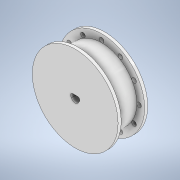
# Autodesk Inventor part: WinderSpoolTraditionalMachining
Saved by Autodesk Inventor 2021 (Build 250183000, 183)
## iProperties
Created: 2020-03-14
Part Number: WinderSpoolTraditionalMachining
Material: Generic
Document SubType Name: Modeling
Designer: elmar
Density: 1 g/cm^3
Appearance: White
Author: elmar
Autodesk Inventor part; units mm, degrees
ref_plane "YZ Plane" through (0, 0, 0) normal (1, 0, 0) x (0, 1, 0)
ref_plane "XZ Plane" through (0, 0, 0) normal (0, 1, 0) x (-1, 0, 0)
ref_plane "XY Plane" through (0, 0, 0) normal (0, 0, 1) x (1, 0, 0)
sketch "Sketch1" plane through (0, 0, 0) normal (0, 0, 1) x (1, 0, 0)
  circle A0 centre (0, 0) radius 22.5
  dimension "d0" = 45
  constraints: 1 centre point, 1 coincident
  measures "d0" diameter of A0
extrude "Extrusion1" add sketch "Sketch1" along normal mid plane 19
sketch "Sketch2" plane through (0, 0, 9.5) normal (0, 0, 1) x (1, 0, 0)
  circle A0 centre (0, 0) radius 27.5
  circle A1 centre (0, 0) radius 22.5 projected
  dimension "d3" = 5
  constraints: 1 centre point, 1 coincident
  measures "d3" radial gap between concentric circles of A0 A1
extrude "Extrusion2" add sketch "Sketch2" against normal blind 2 contours A0 | A1
sketch "Sketch3" plane through (0, 0, -9.5) normal (0, 0, -1) x (-1, 0, 0)
  circle A0 centre (0, 0) radius 27.5 projected
  circle A1 centre (0, 0) radius 22.5 projected
extrude "Extrusion3" add sketch "Sketch3" against normal blind 2
sketch "Sketch4" plane through (0, 0, 9.5) normal (0, 0, 1) x (1, 0, 0)
  circle A0 centre (0, 0) radius 2.5
  line L0 (-1.5, 2) -> (1.5, 2)
  circle A1 centre (-1.5, 0.5) radius 1.5
  line L1 (0, 38.5) -> (0, -38.5) projected
  circle A2 centre (1.5, 0.5) radius 1.5
  point P0 (2.4, -0.7)
  point P1 (1.5, 2)
  point P2 (-2.4, -0.7)
  dimension "d25" = 3
  dimension "d8" = 5
  dimension "d9" = 4.5
  constraints: 2 centre point, 2 end point, 2 horizontal, 2 point on circle, 1 coincident, 1 symmetric about line, 1 tangent, 3 other
  measures "d8" diameter of A0
extrude "Extrusion4" cut sketch "Sketch4" against normal through all contours A0 A2 | A0 A2 | A2 L1 L0 | A0 L1 A2 | L1 A1 L0 | A1 A0 | L1 A0 A1 | A0 A1
sketch "Sketch5" plane through (0, 0, -7.5) normal (0, 0, 1) x (1, 0, 0)
  line L0 (0, -38.5) -> (0, 38.5) projected
  circle A0 centre (0, 24) radius 1.5
  circle A1 centre (0, 0) radius 22.5 projected
  dimension "d31" = 3
  constraints: 1 centre point, 1 point on line, 1 tangent
  measures "d31" diameter of A0
extrude "Extrusion5" cut sketch "Sketch5" against normal through all contours A0 L0 | L0 A0
pattern_circular "Circular Pattern1" count 12 over 360 about axis through (0, 0, -10) along (0, 0, 1) of "Extrusion5"
